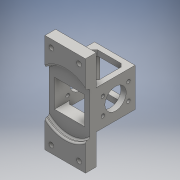
# Autodesk Inventor part: base_plate_new
Saved by Autodesk Inventor 2016 (Build 200138000, 138)
## iProperties
Created: 2016-02-09
Part Number: base_plate_new
Material: Generic
Document SubType Name: Modeling
Designer: element
Density: 1 g/cm^3
Appearance: Default
Mass: 40.9729 g
Surface Area: 180.391 cm^2
Volume: 40.9729 cm^3
Author: element
Autodesk Inventor part; units mm, degrees
ref_plane "YZ Plane" through (0, 0, 0) normal (1, 0, 0) x (0, 1, 0)
ref_plane "XZ Plane" through (0, 0, 0) normal (0, 1, 0) x (-1, 0, 0)
ref_plane "XY Plane" through (0, 0, 0) normal (0, 0, 1) x (1, 0, 0)
sketch "Sketch1" plane through (0, 0, 0) normal (0, 1, 0) x (-1, 0, 0)
  line L0 (0, 0) -> (19, 0)
  line L1 (0, 0) -> (-19, 0)
  line L2 (19, 0) -> (19, 46.5)
  line L3 (-19, 0) -> (-19, 46.5)
  line L4 (19, 46.5) -> (-19, 46.5)
  dimension "d0" = 19
  dimension "d1" = 19
  dimension "d2" = 46.5
  dimension "d5" = 46.5
  constraints: 10 end point, 2 horizontal, 2 vertical
  measures "d0" distance of L0.start L0.end
  measures "d1" distance of L0.start L1.end
  measures "d2" distance of L0.end L2.end
  measures "d5" distance of L1.end L3.end
sketch "Sketch2" plane through (0, 0, 0) normal (0, 1, 0) x (-1, 0, 0)
  circle A0 centre (0, 0) radius 28
  line L0 (14, 13) -> (-14, 13)
  line L1 (-14, 13) -> (-14, -13)
  line L2 (-14, -13) -> (14, -13)
  line L3 (14, -13) -> (14, 13)
  dimension "d7" = 56
  dimension "d215" = 14
  dimension "d216" = 28
  dimension "d217" = 26
  dimension "d218" = 13
  constraints: 8 end point, 2 parallel, 1 centre point, 1 coincident, 1 horizontal, 1 perpendicular
  measures "d7" diameter of A0
  measures "d215" distance from line of point (0, 0) L3
  measures "d216" distance between parallel lines of L1 L3
  measures "d217" distance between parallel lines of L2 L0
  measures "d218" distance from line of point (0, 0) L0
extrude "Extrusion1" add sketch "Sketch1" along normal blind 10
extrude "Extrusion2" cut sketch "Sketch2" along normal blind 4 contours A0 | L3 L2 L1 L0
sketch "Sketch3" plane through (0, 0, 0) normal (0, 1, 0) x (-1, 0, 0)
  line L0 (0, 0) -> (13, 0)
  line L1 (13, 0) -> (13, 39.5)
  line L2 (0, 0) -> (-13, 0)
  line L3 (-13, 0) -> (-13, 39.5)
  circle A0 centre (13, 39.5) radius 2.25
  circle A1 centre (-13, 39.5) radius 2.25
  dimension "d8" = 13
  dimension "d9" = 39.5
  dimension "d11" = 13
  dimension "d13" = 39.5
  dimension "d14" = 4.5
  dimension "d15" = 4.5
  constraints: 8 end point, 4 coincident, 2 centre point, 2 horizontal, 1 perpendicular, 1 vertical
  measures "d8" distance of L0.start L0.end
  measures "d9" distance of L0.end L1.end
  measures "d11" distance of L0.start L2.end
  measures "d13" distance of L2.end L3.end
  measures "d14" diameter of A0
  measures "d15" diameter of A1
hole "Hole2" at (-13, 0, 39.5) direction (0, 1, 0) diameter 4.5 end through all
hole "Hole3" at (13, 0, 39.5) direction (0, 1, 0) diameter 4.5 end through all
sketch "Sketch4" plane through (0, 10, 0) normal (0, 1, 0) x (1, 0, 0)
  line L0 (0, 0) -> (-13, 0)
  line L1 (19, 0) -> (-19, 0) projected
  line L2 (-13, 0) -> (-13, -39.5)
  line L3 (0, 0) -> (13, 0)
  line L4 (13, 0) -> (13, -39.5)
  line L5 (-13, -35.2565) -> (-9.325, -37.3782)
  line L6 (-9.325, -37.3782) -> (-9.325, -41.6218)
  line L7 (-9.325, -41.6218) -> (-13, -43.7435)
  line L8 (-13, -43.7435) -> (-16.675, -41.6218)
  line L9 (-16.675, -41.6218) -> (-16.675, -37.3782)
  line L10 (-16.675, -37.3782) -> (-13, -35.2565)
  line L11 (13, -35.2565) -> (16.675, -37.3782)
  line L12 (16.675, -37.3782) -> (16.675, -41.6218)
  line L13 (16.675, -41.6218) -> (13, -43.7435)
  line L14 (13, -43.7435) -> (9.325, -41.6218)
  line L15 (9.325, -41.6218) -> (9.325, -37.3782)
  line L16 (9.325, -37.3782) -> (13, -35.2565)
  dimension "d59" = 13
  dimension "d60" = 39.5
  dimension "d61" = 39.5
  dimension "d62" = 13
  dimension "d63" = 7.35
  dimension "d64" = 7.35
  constraints: 32 end point, 4 point on line, 2 coincident, 2 vertical, 26 other
  measures "d59" distance of L0.start L0.end
  measures "d60" distance of L0.end L2.end
  measures "d61" distance of L3.end L4.end
  measures "d62" distance from line of L0.start L4
  measures "d63" distance between parallel lines of L6 L9
  measures "d64" distance between parallel lines of L12 L15
extrude "Extrusion3" cut sketch "Sketch4" against normal blind 4 contours L5 L6 L7 L8 L9 L10
extrude "Extrusion4" cut sketch "Sketch4" against normal blind 4 contours L11 L12 L13 L14 L15 L16
mirror "Mirror5" about plane through (0, 0, 0) normal (0, 0, 1) of "Extrusion4", "Extrusion3", "Hole3", "Hole2", "Extrusion2", "Extrusion1"
fillet "Fillet10" radius 1.5 4 edges at (0, 0, 28) (0, 0, -28) (0, 4, 28) (0, 4, -28)
sketch "Sketch5" plane through (0, 10, 0) normal (0, 1, 0) x (1, 0, 0)
  line L0 (0, 0) -> (0, -13)
  line L1 (0, -18) -> (-19, -18)
  line L2 (-19, -46.5) -> (-19, 46.5) projected
  line L3 (-19, -18) -> (-19, -13)
  line L4 (-19, -13) -> (0, -13)
  line L5 (0, -13) -> (19, -13)
  line L6 (19, -13) -> (19, -18)
  line L7 (19, -18) -> (0, -18)
  point P0 (-19, -45)
  point P1 (-19, 45)
  dimension "d73" = 13
  dimension "d75" = 19
  dimension "d76" = 19
  dimension "d77" = 5
  constraints: 14 end point, 5 perpendicular, 1 horizontal, 1 point on line, 1 vertical
  measures "d73" distance of L0.start L0.end
  measures "d75" distance of L3.end L0.end
  measures "d76" distance of L0.end L5.end
  measures "d77" distance between parallel lines of L4 L1
extrude "Extrusion5" add sketch "Sketch5" along normal blind 36.5
mirror "Mirror7" about plane through (0, 0, 0) normal (0, 0, 1) of "Extrusion5"
sketch "Sketch7" plane through (19, 10, -18) normal (0, 0, -1) x (-1, 0, 0)
  line L0 (0, 0) -> (0, 36.5) projected
  line L1 (0, 0) -> (0, 36.5)
  line L2 (0, 36.5) -> (5, 36.5)
  line L3 (38, 36.5) -> (0, 36.5) projected
  line L4 (0, 0) -> (5.1907, 0)
  line L5 (0, 0) -> (0, 36.5) projected
  line L6 (0, 0) -> (5, 0)
  line L7 (38, 0) -> (0, 0) projected
  line L8 (5, 0) -> (5, 36.5)
  line L9 (5, 0) -> (33, 0)
  line L10 (33, 0) -> (33, 36.5)
  line L11 (33, 36.5) -> (38, 36.5)
  line L12 (38, 36.5) -> (38, 0)
  line L13 (33, 0) -> (38, 0)
  point P0 (19, -10)
  dimension "d96" = 5
  dimension "d97" = 5
  dimension "d98" = 28
  constraints: 20 end point, 6 point on line, 3 perpendicular, 1 collinear, 1 horizontal
  measures "d96" distance of L0.end L2.end
  measures "d97" distance between parallel lines of L10 L12
  measures "d98" distance between parallel lines of L8 L10
extrude "Extrusion7" add sketch "Sketch7" against normal blind 35 contours L0 L2 L8 L4 | L3 L12 L7 L10
sketch "Sketch9" plane through (19, 0, 46.5) normal (1, 0, 0) x (0, 0, -1)
  line L0 (46.5, 0) -> (46.5, 16.25)
  circle A0 centre (38.5, 40.25) radius 1.7
  circle A1 centre (38.5, 16.25) radius 1.7
  circle A2 centre (54.5, 40.25) radius 1.7
  circle A3 centre (54.5, 16.25) radius 1.7
  line L1 (46.5, 16.25) -> (54.5, 16.25)
  line L2 (46.5, 16.25) -> (38.5, 16.25)
  line L3 (38.5, 40.25) -> (54.5, 40.25)
  line L4 (54.5, 40.25) -> (54.5, 16.25)
  line L5 (38.5, 28.25) -> (46.5, 28.25)
  line L6 (46.5, 28.25) -> (46.5, 16.25)
  line L7 (38.5, 16.25) -> (38.5, 28.25)
  line L8 (38.5, 28.25) -> (38.5, 40.25)
  circle A4 centre (46.5, 28.25) radius 10
  point P0 (27, 46.5)
  dimension "d172" = 3.4
  dimension "d173" = 3.4
  dimension "d174" = 3.4
  dimension "d175" = 3.4
  dimension "d176" = 16.25
  dimension "d177" = 8
  dimension "d178" = 8
  dimension "d179" = 12
  dimension "d180" = 12
  dimension "d181" = 20
  constraints: 18 end point, 6 coincident, 5 centre point, 3 horizontal, 2 perpendicular, 2 vertical, 1 collinear
  measures "d172" diameter of A0
  measures "d173" diameter of A2
  measures "d174" diameter of A3
  measures "d175" diameter of A1
  measures "d176" distance of L0.start L0.end
  measures "d177" distance of L0.end L2.end
  measures "d178" distance of L0.end L1.end
  measures "d179" distance between parallel lines of L2 L5
  measures "d180" distance of L5.start L3.start
  measures "d181" diameter of A4
hole "Hole11" at (19, 40.25, 8) at (19, 40.25, -8) at (19, 16.25, -8) at (19, 16.25, 8) direction (-1, 0, 0) diameter 3.4 end through all
hole "Hole12" at (19, 28.25, 0) direction (-1, 0, 0) diameter 20 end through all
sketch "Sketch10" plane through (-19, 46.5, 18) normal (0, 0, 1) x (1, 0, 0)
  line L0 (0, -36.5) -> (0, 0) projected
  line L1 (0, 0) -> (19, 0)
  line L2 (33, 0) -> (5, 0) projected
  line L3 (5, -31.5) -> (33, -31.5)
  line L4 (33, -31.5) -> (33, -5)
  line L5 (33, -5) -> (5, -5)
  line L6 (5, -5) -> (5, -31.5)
  line L7 (0, -36.5) -> (38, -36.5) projected
  line L8 (38, -36.5) -> (38, 0) projected
  point P0 (19, -46.5)
  point P1 (0, -33.5)
  dimension "d206" = 5
  dimension "d207" = 5
  dimension "d208" = 5
  dimension "d209" = 5
  constraints: 10 end point, 2 parallel, 1 horizontal, 1 midpoint, 1 perpendicular
  measures "d206" distance between parallel lines of L0 L6
  measures "d207" distance between parallel lines of L7 L3
  measures "d208" distance between parallel lines of L8 L4
  measures "d209" distance between parallel lines of L1 L5
extrude "Extrusion9" cut sketch "Sketch10" against normal blind 50
chamfer "Chamfer9" distance 3 angle 45 8 edges at (-14, 15, 15.5) (14, 15, 15.5) (14, 15, -15.5) (-14, 15, -15.5) (-14, 41.5, 15.5) (-14, 41.5, -15.5) (14, 41.5, 15.5) (14, 41.5, -15.5)
extrude "Extrusion10" cut sketch "Sketch2" along normal blind 10 contours L3 L2 L1 L0
equation "\"d1\" = d0"
equation "\"d5\" = d2"
equation "\"d11\" = d8"
equation "\"d13\" = d9"
equation "\"d15\" = d14"
equation "\"d27\" = d14"
equation "\"d34\" = d15"
equation "\"d59\" = d8"
equation "\"d60\" = d9"
equation "\"d61\" = d9"
equation "\"d62\" = d8"
equation "\"d64\" = d63"
equation "\"d76\" = d75"
body "Solid1"
